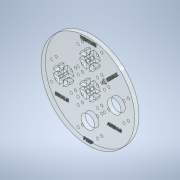
# Autodesk Inventor part: Top_Plate_For_Valve
Saved by Autodesk Inventor 2020 (Build 240168000, 168)
## iProperties
Created: 2021-06-26
Part Number: Top_Plate_For_Valve
Material: Glass
Document SubType Name: Modeling
Designer: Workshop
Density: 2.18 g/cm^3
Appearance: Clear
Author: Workshop
Autodesk Inventor part; units mm, degrees
ref_plane "YZ Plane" through (0, 0, 0) normal (1, 0, 0) x (0, 1, 0)
ref_plane "XZ Plane" through (0, 0, 0) normal (0, 1, 0) x (-1, 0, 0)
ref_plane "XY Plane" through (0, 0, 0) normal (0, 0, 1) x (1, 0, 0)
sketch "Sketch1" plane through (0, 0, 0) normal (0, 0, 1) x (1, 0, 0)
  circle A0 centre (0, -30.9758) radius 8 projected
  circle A1 centre (42.3779, -11.4021) radius 1.5 projected
  circle A2 centre (11.4021, -19.5736) radius 1.5 projected
  circle A3 centre (-11.4021, -19.5737) radius 1.5 projected
  circle A4 centre (-11.4021, -42.3779) radius 1.5 projected
  circle A5 centre (11.4021, -42.3778) radius 1.5 projected
  circle A6 centre (19.5737, -11.4021) radius 1.5 projected
  circle A7 centre (42.3778, 11.4021) radius 1.5 projected
  circle A8 centre (19.5736, 11.4021) radius 1.5 projected
  circle A9 centre (-19.5736, -11.4021) radius 1.5 projected
  circle A10 centre (-11.4021, 11.4021) radius 1.5 projected
  circle A11 centre (0, 0) radius 55 projected
  circle A12 centre (-42.3778, -11.4021) radius 1.5 projected
  circle A13 centre (-11.4021, 19.5736) radius 1.5 projected
  circle A14 centre (11.4021, 19.5737) radius 1.5 projected
  circle A15 centre (-19.5737, 11.4021) radius 1.5 projected
  circle A16 centre (-42.3779, 11.4021) radius 1.5 projected
  line L0 (-3.5186, 28.9238) -> (-9.6538, 28.9238) projected
  arc A17 (-9.6538, 28.9238) -> (-2.019, 21.3151) centre (0, 30.9758) ccw projected
  line L1 (-2.019, 21.3151) -> (-2.0129, 27.4347) projected
  arc A18 (-3.5186, 28.9238) -> (-2.0129, 27.4347) centre (0, 30.9758) ccw projected
  line L2 (3.5186, 28.9238) -> (9.6538, 28.9238) projected
  arc A19 (2.019, 21.3151) -> (9.6538, 28.9238) centre (0, 30.9758) ccw projected
  line L3 (2.019, 21.3151) -> (2.0129, 27.4347) projected
  arc A20 (2.0129, 27.4347) -> (3.5186, 28.9238) centre (0, 30.9758) ccw projected
  line L4 (-3.5186, 33.0277) -> (-9.6538, 33.0277) projected
  arc A21 (-2.019, 40.6365) -> (-9.6538, 33.0277) centre (0, 30.9758) ccw projected
  line L5 (-2.019, 40.6365) -> (-2.0129, 34.5169) projected
  arc A22 (-2.0129, 34.5169) -> (-3.5186, 33.0277) centre (0, 30.9758) ccw projected
  line L6 (3.5186, 33.0277) -> (9.6538, 33.0277) projected
  arc A23 (9.6538, 33.0277) -> (2.019, 40.6365) centre (0, 30.9758) ccw projected
  line L7 (2.019, 40.6365) -> (2.0129, 34.5169) projected
  arc A24 (3.5186, 33.0277) -> (2.0129, 34.5169) centre (0, 30.9758) ccw projected
  circle A25 centre (0, 30.9758) radius 2.25 projected
  circle A26 centre (11.4021, 42.3779) radius 1.5 projected
  circle A27 centre (-11.4021, 42.3778) radius 1.5 projected
  line L8 (-2.052, 3.5186) -> (-2.052, 9.6538) projected
  arc A28 (-2.052, 9.6538) -> (-9.6607, 2.019) centre (0, 0) ccw projected
  line L9 (-9.6607, 2.019) -> (-3.5411, 2.0129) projected
  arc A29 (-2.052, 3.5186) -> (-3.5411, 2.0129) centre (0, 0) ccw projected
  circle A30 centre (0, 0) radius 2.25 projected
  line L10 (-2.052, -3.5186) -> (-2.052, -9.6538) projected
  arc A31 (-9.6607, -2.019) -> (-2.052, -9.6538) centre (0, 0) ccw projected
  line L11 (-9.6607, -2.019) -> (-3.5411, -2.0129) projected
  arc A32 (-3.5411, -2.0129) -> (-2.052, -3.5186) centre (0, 0) ccw projected
  circle A33 centre (-11.4021, -11.4021) radius 1.5 projected
  line L12 (-33.0277, -3.5186) -> (-33.0277, -9.6538) projected
  arc A34 (-40.6365, -2.019) -> (-33.0277, -9.6538) centre (-30.9758, 0) ccw projected
  line L13 (-40.6365, -2.019) -> (-34.5169, -2.0129) projected
  arc A35 (-34.5169, -2.0129) -> (-33.0277, -3.5186) centre (-30.9758, 0) ccw projected
  line L14 (-33.0277, 3.5186) -> (-33.0277, 9.6538) projected
  arc A36 (-33.0277, 9.6538) -> (-40.6365, 2.019) centre (-30.9758, 0) ccw projected
  line L15 (-40.6365, 2.019) -> (-34.5169, 2.0129) projected
  arc A37 (-33.0277, 3.5186) -> (-34.5169, 2.0129) centre (-30.9758, 0) ccw projected
  line L16 (2.052, 3.5186) -> (2.052, 9.6538) projected
  arc A38 (9.6607, 2.019) -> (2.052, 9.6538) centre (0, 0) ccw projected
  line L17 (9.6607, 2.019) -> (3.5411, 2.0129) projected
  arc A39 (3.5411, 2.0129) -> (2.052, 3.5186) centre (0, 0) ccw projected
  line L18 (2.052, -3.5186) -> (2.052, -9.6538) projected
  arc A40 (2.052, -9.6538) -> (9.6607, -2.019) centre (0, 0) ccw projected
  line L19 (9.6607, -2.019) -> (3.5411, -2.0129) projected
  arc A41 (2.052, -3.5186) -> (3.5411, -2.0129) centre (0, 0) ccw projected
  line L20 (-28.9238, 3.5186) -> (-28.9238, 9.6538) projected
  arc A42 (-21.3151, 2.019) -> (-28.9238, 9.6538) centre (-30.9758, 0) ccw projected
  line L21 (-21.3151, 2.019) -> (-27.4347, 2.0129) projected
  arc A43 (-27.4347, 2.0129) -> (-28.9238, 3.5186) centre (-30.9758, 0) ccw projected
  line L22 (-28.9238, -3.5186) -> (-28.9238, -9.6538) projected
  arc A44 (-28.9238, -9.6538) -> (-21.3151, -2.019) centre (-30.9758, 0) ccw projected
  line L23 (-21.3151, -2.019) -> (-27.4347, -2.0129) projected
  arc A45 (-28.9238, -3.5186) -> (-27.4347, -2.0129) centre (-30.9758, 0) ccw projected
  circle A46 centre (-30.9758, 0) radius 1.5 projected
  circle A47 centre (11.4021, 11.4021) radius 1.5 projected
  circle A48 centre (30.9758, 0) radius 8 projected
  circle A49 centre (11.4021, -11.4021) radius 1.5 projected
  point P0 (0, 0)
extrude "Extrusion1" add sketch "Sketch1" along normal mid plane 5
sketch "Sketch2" plane through (0, 0, 2.5) normal (0, 0, 1) x (1, 0, 0)
  line L0 (-9.3534, 52.1011) -> (9.3534, 52.1011) construction
  line L1 (9.3534, 52.1011) -> (9.3534, 49) construction
  line L2 (9.3534, 49) -> (-9.3534, 49) construction
  line L3 (-9.3534, 49) -> (-9.3534, 52.1011) construction
  line L4 (-38.9076, -20) -> (-23.0439, -20) construction
  line L5 (-23.0439, -20) -> (-23.0439, -23.05) construction
  line L6 (-23.0439, -23.05) -> (-38.9076, -23.05) construction
  line L7 (-38.9076, -23.05) -> (-38.9076, -20) construction
  line L8 (22.3314, -20) -> (39.6201, -20) construction
  line L9 (39.6201, -20) -> (39.6201, -23.05) construction
  line L10 (39.6201, -23.05) -> (22.3314, -23.05) construction
  line L11 (22.3314, -23.05) -> (22.3314, -20) construction
  line L12 (-5.6862, -49) -> (5.6862, -49) construction
  line L13 (5.6862, -49) -> (5.6862, -52.05) construction
  line L14 (5.6862, -52.05) -> (-5.6862, -52.05) construction
  line L15 (-5.6862, -52.05) -> (-5.6862, -49) construction
  line L16 (20.842, 22.9986) -> (33.067, 35.2236) construction
  line L17 (33.067, 35.2236) -> (35.2236, 33.067) construction
  line L18 (35.2236, 33.067) -> (22.9986, 20.842) construction
  line L19 (22.9986, 20.842) -> (20.842, 22.9986) construction
  circle A0 centre (-30.9758, 0) radius 1.5 projected
  circle A1 centre (30.9758, 0) radius 8 projected
  circle A2 centre (0, 0) radius 2.25 projected
  line L20 (0, 0) -> (21.9203, 21.9203) construction
  line L21 (0, 0) -> (31, 0) construction
  line L22 (-8.2631, 49.0511) -> (-9.3534, 52.1011)
  line L23 (-9.3534, 52.1011) -> (-8.6862, 52.1011)
  line L24 (-8.6862, 52.1011) -> (-7.9121, 49.8439)
  line L25 (-7.9121, 49.8439) -> (-7.1659, 52.1011)
  line L26 (-7.1659, 52.1011) -> (-6.5126, 52.1011)
  line L27 (-6.5126, 52.1011) -> (-7.6029, 49.0511)
  line L28 (-7.6029, 49.0511) -> (-8.2631, 49.0511)
  line L29 (-6.1988, 49.0511) -> (-6.1988, 52.1011)
  line L30 (-6.1988, 52.1011) -> (-3.9369, 52.1011)
  line L31 (-3.9369, 52.1011) -> (-3.9369, 51.5851)
  line L32 (-3.9369, 51.5851) -> (-5.5828, 51.5851)
  line L33 (-5.5828, 51.5851) -> (-5.5828, 50.9086)
  line L34 (-5.5828, 50.9086) -> (-4.0508, 50.9086)
  line L35 (-4.0508, 50.9086) -> (-4.0508, 50.3925)
  line L36 (-4.0508, 50.3925) -> (-5.5828, 50.3925)
  line L37 (-5.5828, 50.3925) -> (-5.5828, 49.5672)
  line L38 (-5.5828, 49.5672) -> (-3.8788, 49.5672)
  line L39 (-3.8788, 49.5672) -> (-3.8788, 49.0511)
  line L40 (-3.8788, 49.0511) -> (-6.1988, 49.0511)
  line L41 (-3.351, 49.0511) -> (-3.351, 52.1011)
  line L42 (-3.351, 52.1011) -> (-2.7536, 52.1011)
  line L43 (-2.7536, 52.1011) -> (-1.5006, 50.0554)
  line L44 (-1.5006, 50.0554) -> (-1.5006, 52.1011)
  line L45 (-1.5006, 52.1011) -> (-0.931, 52.1011)
  line L46 (-0.931, 52.1011) -> (-0.931, 49.0511)
  line L47 (-0.931, 49.0511) -> (-1.5471, 49.0511)
  line L48 (-1.5471, 49.0511) -> (-2.7815, 51.0527)
  line L49 (-2.7815, 51.0527) -> (-2.7815, 49.0511)
  line L50 (-2.7815, 49.0511) -> (-3.351, 49.0511)
  line L51 (0.408, 49.0511) -> (0.408, 51.5851)
  line L52 (0.408, 51.5851) -> (-0.4963, 51.5851)
  line L53 (-0.4963, 51.5851) -> (-0.4963, 52.1011)
  line L54 (-0.4963, 52.1011) -> (1.926, 52.1011)
  line L55 (1.926, 52.1011) -> (1.926, 51.5851)
  line L56 (1.926, 51.5851) -> (1.024, 51.5851)
  line L57 (1.024, 51.5851) -> (1.024, 49.0511)
  line L58 (1.024, 49.0511) -> (0.408, 49.0511)
  line L59 (2.3212, 52.1011) -> (2.9373, 52.1011)
  line L60 (2.9373, 52.1011) -> (2.9373, 50.4483)
  spline S0 degree 2 poles (2.9373, 50.4483) (2.9373, 50.0554) (2.9605, 49.9392) knots 0 0 0 1 1 1
  spline S1 degree 2 poles (2.9605, 49.9392) (3, 49.7532) (3.2976, 49.5254) (3.5556, 49.5254) knots 0 0 0 1 2 2 2
  spline S2 degree 2 poles (3.5556, 49.5254) (3.816, 49.5254) (4.0833, 49.7393) (4.1368, 50.0508) (4.1368, 50.4134) knots 0 0 0 1 2 3 3 3
  line L61 (4.1368, 50.4134) -> (4.1368, 52.1011)
  line L62 (4.1368, 52.1011) -> (4.7528, 52.1011)
  line L63 (4.7528, 52.1011) -> (4.7528, 50.4994)
  spline S3 degree 2 poles (4.7528, 50.4994) (4.7528, 49.9508) (4.6529, 49.4975) (4.3855, 49.186) (3.9345, 49) (3.5742, 49) knots 0 0 0 1 2 3 4 4 4
  spline S4 degree 2 poles (3.5742, 49) (3.1372, 49) (2.6862, 49.2022) (2.4235, 49.5231) (2.3817, 49.7021) knots 0 0 0 1 2 3 3 3
  spline S5 degree 2 poles (2.3817, 49.7021) (2.3212, 49.9624) (2.3212, 50.4739) knots 0 0 0 1 1 1
  line L64 (2.3212, 50.4739) -> (2.3212, 52.1011)
  line L65 (5.4038, 49.0511) -> (5.4038, 52.1011)
  line L66 (5.4038, 52.1011) -> (6.7009, 52.1011)
  spline S6 degree 2 poles (6.7009, 52.1011) (7.1914, 52.1011) (7.6331, 51.9361) (7.9005, 51.5176) (7.9005, 51.2457) knots 0 0 0 1 2 3 3 3
  spline S7 degree 2 poles (7.9005, 51.2457) (7.9005, 50.9039) (7.4983, 50.4553) (7.0961, 50.3971) knots 0 0 0 1 2 2 2
  spline S8 degree 2 poles (7.0961, 50.3971) (7.2961, 50.2809) (7.5564, 50.0019) (7.7773, 49.6463) knots 0 0 0 1 2 2 2
  line L67 (7.7773, 49.6463) -> (8.1492, 49.0511)
  line L68 (8.1492, 49.0511) -> (7.4123, 49.0511)
  line L69 (7.4123, 49.0511) -> (6.9683, 49.716)
  spline S9 degree 2 poles (6.9683, 49.716) (6.7288, 50.0717) (6.5545, 50.2577) (6.3592, 50.3251) (6.1453, 50.3251) knots 0 0 0 1 2 3 3 3
  line L70 (6.1453, 50.3251) -> (6.0198, 50.3251)
  line L71 (6.0198, 50.3251) -> (6.0198, 49.0511)
  line L72 (6.0198, 49.0511) -> (5.4038, 49.0511)
  line L73 (6.0198, 50.8109) -> (6.4754, 50.8109)
  spline S10 degree 2 poles (6.4754, 50.8109) (6.9195, 50.8109) (7.1403, 50.8853) (7.2658, 51.069) (7.2658, 51.2061) knots 0 0 0 1 2 3 3 3
  spline S11 degree 2 poles (7.2658, 51.2061) (7.2658, 51.3596) (7.1008, 51.5502) (6.952, 51.5758) knots 0 0 0 1 2 2 2
  spline S12 degree 2 poles (6.952, 51.5758) (6.8753, 51.5851) (6.501, 51.5851) knots 0 0 0 1 1 1
  line L74 (6.501, 51.5851) -> (6.0198, 51.5851)
  line L75 (6.0198, 51.5851) -> (6.0198, 50.8109)
  line L76 (8.4607, 49.0511) -> (8.4607, 52.1011)
  line L77 (8.4607, 52.1011) -> (9.0768, 52.1011)
  line L78 (9.0768, 52.1011) -> (9.0768, 49.0511)
  line L79 (9.0768, 49.0511) -> (8.4607, 49.0511)
  line L80 (23.2189, 21.0622) -> (21.0622, 23.2189)
  line L81 (21.0622, 23.2189) -> (22.6617, 24.8183)
  line L82 (22.6617, 24.8183) -> (23.0266, 24.4534)
  line L83 (23.0266, 24.4534) -> (21.8628, 23.2896)
  line L84 (21.8628, 23.2896) -> (22.3411, 22.8113)
  line L85 (22.3411, 22.8113) -> (23.4244, 23.8945)
  line L86 (23.4244, 23.8945) -> (23.7893, 23.5296)
  line L87 (23.7893, 23.5296) -> (22.7061, 22.4463)
  line L88 (22.7061, 22.4463) -> (23.2896, 21.8628)
  line L89 (23.2896, 21.8628) -> (24.4945, 23.0677)
  line L90 (24.4945, 23.0677) -> (24.8594, 22.7028)
  line L91 (24.8594, 22.7028) -> (23.2189, 21.0622)
  line L92 (25.0107, 22.854) -> (24.6326, 24.7214)
  line L93 (24.6326, 24.7214) -> (22.923, 25.0797)
  line L94 (22.923, 25.0797) -> (23.431, 25.5876)
  line L95 (23.431, 25.5876) -> (24.5027, 25.3707)
  line L96 (24.5027, 25.3707) -> (24.2857, 26.4424)
  line L97 (24.2857, 26.4424) -> (24.7937, 26.9504)
  line L98 (24.7937, 26.9504) -> (25.1471, 25.2392)
  line L99 (25.1471, 25.2392) -> (27.0161, 24.8594)
  line L100 (27.0161, 24.8594) -> (26.4901, 24.3334)
  line L101 (26.4901, 24.3334) -> (25.2819, 24.5849)
  line L102 (25.2819, 24.5849) -> (25.5334, 23.3767)
  line L103 (25.5334, 23.3767) -> (25.0107, 22.854)
  line L104 (27.2397, 25.083) -> (25.083, 27.2397)
  line L105 (25.083, 27.2397) -> (25.5186, 27.6753)
  line L106 (25.5186, 27.6753) -> (26.3668, 26.8271)
  line L107 (26.3668, 26.8271) -> (27.2199, 27.6802)
  line L108 (27.2199, 27.6802) -> (26.3717, 28.5284)
  line L109 (26.3717, 28.5284) -> (26.8074, 28.964)
  line L110 (26.8074, 28.964) -> (28.964, 26.8074)
  line L111 (28.964, 26.8074) -> (28.5284, 26.3717)
  line L112 (28.5284, 26.3717) -> (27.5849, 27.3153)
  line L113 (27.5849, 27.3153) -> (26.7317, 26.4622)
  line L114 (26.7317, 26.4622) -> (27.6753, 25.5186)
  line L115 (27.6753, 25.5186) -> (27.2397, 25.083)
  line L116 (31.3591, 29.2024) -> (30.8856, 28.729)
  line L117 (30.8856, 28.729) -> (30.2084, 29.0314)
  line L118 (30.2084, 29.0314) -> (29.347, 28.1701)
  line L119 (29.347, 28.1701) -> (29.6577, 27.501)
  line L120 (29.6577, 27.501) -> (29.1958, 27.0391)
  line L121 (29.1958, 27.0391) -> (27.8775, 30.0341)
  line L122 (27.8775, 30.0341) -> (28.341, 30.4977)
  line L123 (28.341, 30.4977) -> (31.3591, 29.2024)
  line L124 (29.7037, 29.2566) -> (28.6073, 29.758)
  line L125 (28.6073, 29.758) -> (29.1136, 28.6665)
  line L126 (29.1136, 28.6665) -> (29.7037, 29.2566)
  line L127 (31.604, 29.4473) -> (29.4654, 31.5859)
  line L128 (29.4654, 31.5859) -> (29.901, 32.0215)
  line L129 (29.901, 32.0215) -> (31.6747, 30.2478)
  line L130 (31.6747, 30.2478) -> (32.7579, 31.3311)
  line L131 (32.7579, 31.3311) -> (33.1229, 30.9662)
  line L132 (33.1229, 30.9662) -> (31.604, 29.4473)
  line L133 (33.4335, 31.2769) -> (31.2769, 33.4335)
  line L134 (31.2769, 33.4335) -> (32.8763, 35.033)
  line L135 (32.8763, 35.033) -> (33.2412, 34.668)
  line L136 (33.2412, 34.668) -> (32.0774, 33.5042)
  line L137 (32.0774, 33.5042) -> (32.5557, 33.0259)
  line L138 (32.5557, 33.0259) -> (33.639, 34.1091)
  line L139 (33.639, 34.1091) -> (34.0039, 33.7442)
  line L140 (34.0039, 33.7442) -> (32.9207, 32.6609)
  line L141 (32.9207, 32.6609) -> (33.5042, 32.0774)
  line L142 (33.5042, 32.0774) -> (34.7091, 33.2823)
  line L143 (34.7091, 33.2823) -> (35.0741, 32.9174)
  line L144 (35.0741, 32.9174) -> (33.4335, 31.2769)
  line L145 (25.3907, -23.1011) -> (24.7212, -23.1011)
  line L146 (24.7212, -23.1011) -> (24.4562, -22.4084)
  line L147 (24.4562, -22.4084) -> (23.238, -22.4084)
  line L148 (23.238, -22.4084) -> (22.9846, -23.1011)
  line L149 (22.9846, -23.1011) -> (22.3314, -23.1011)
  line L150 (22.3314, -23.1011) -> (23.517, -20.0511)
  line L151 (23.517, -20.0511) -> (24.1725, -20.0511)
  line L152 (24.1725, -20.0511) -> (25.3907, -23.1011)
  line L153 (24.2586, -21.8923) -> (23.8378, -20.7625)
  line L154 (23.8378, -20.7625) -> (23.424, -21.8923)
  line L155 (23.424, -21.8923) -> (24.2586, -21.8923)
  line L156 (25.6999, -23.1011) -> (25.6999, -20.0511)
  line L157 (25.6999, -20.0511) -> (26.3159, -20.0511)
  line L158 (26.3159, -20.0511) -> (26.3159, -23.1011)
  line L159 (26.3159, -23.1011) -> (25.6999, -23.1011)
  line L160 (26.9041, -23.1011) -> (26.9041, -20.0511)
  line L161 (26.9041, -20.0511) -> (28.2012, -20.0511)
  spline S13 degree 2 poles (28.2012, -20.0511) (28.6918, -20.0511) (29.1334, -20.2162) (29.4008, -20.6346) (29.4008, -20.9066) knots 0 0 0 1 2 3 3 3
  spline S14 degree 2 poles (29.4008, -20.9066) (29.4008, -21.2484) (28.9986, -21.697) (28.5964, -21.7551) knots 0 0 0 1 2 2 2
  spline S15 degree 2 poles (28.5964, -21.7551) (28.7964, -21.8714) (29.0567, -22.1503) (29.2776, -22.506) knots 0 0 0 1 2 2 2
  line L162 (29.2776, -22.506) -> (29.6495, -23.1011)
  line L163 (29.6495, -23.1011) -> (28.9126, -23.1011)
  line L164 (28.9126, -23.1011) -> (28.4686, -22.4363)
  spline S16 degree 2 poles (28.4686, -22.4363) (28.2291, -22.0806) (28.0548, -21.8946) (27.8595, -21.8272) (27.6456, -21.8272) knots 0 0 0 1 2 3 3 3
  line L165 (27.6456, -21.8272) -> (27.5201, -21.8272)
  line L166 (27.5201, -21.8272) -> (27.5201, -23.1011)
  line L167 (27.5201, -23.1011) -> (26.9041, -23.1011)
  line L168 (27.5201, -21.3413) -> (27.9757, -21.3413)
  spline S17 degree 2 poles (27.9757, -21.3413) (28.4198, -21.3413) (28.6406, -21.267) (28.7661, -21.0833) (28.7661, -20.9462) knots 0 0 0 1 2 3 3 3
  spline S18 degree 2 poles (28.7661, -20.9462) (28.7661, -20.7927) (28.6011, -20.6021) (28.4523, -20.5765) knots 0 0 0 1 2 2 2
  spline S19 degree 2 poles (28.4523, -20.5765) (28.3756, -20.5672) (28.0013, -20.5672) knots 0 0 0 1 1 1
  line L169 (28.0013, -20.5672) -> (27.5201, -20.5672)
  line L170 (27.5201, -20.5672) -> (27.5201, -21.3413)
  line L171 (29.982, -20.0511) -> (31.2024, -20.0511)
  spline S20 degree 2 poles (31.2024, -20.0511) (31.5651, -20.0511) (31.9208, -20.1116) (32.202, -20.3022) (32.3903, -20.6207) (32.3903, -20.8183) knots 0 0 0 1 2 3 4 4 4
  spline S21 degree 2 poles (32.3903, -20.8183) (32.3903, -21.0322) (32.1602, -21.3878) (31.9626, -21.4785) knots 0 0 0 1 2 2 2
  spline S22 degree 2 poles (31.9626, -21.4785) (32.2416, -21.5599) (32.5391, -21.9504) (32.5391, -22.2154) knots 0 0 0 1 2 2 2
  spline S23 degree 2 poles (32.5391, -22.2154) (32.5391, -22.4247) (32.3462, -22.8175) (32.0091, -23.0523) (31.765, -23.0802) knots 0 0 0 1 2 3 3 3
  spline S24 degree 2 poles (31.765, -23.0802) (31.6092, -23.0965) (31.0211, -23.1011) knots 0 0 0 1 1 1
  line L172 (31.0211, -23.1011) -> (29.982, -23.1011)
  line L173 (29.982, -23.1011) -> (29.982, -20.0511)
  line L174 (30.598, -21.7691) -> (30.598, -22.5851)
  line L175 (30.598, -22.5851) -> (31.1699, -22.5851)
  spline S25 degree 2 poles (31.1699, -22.5851) (31.5046, -22.5851) (31.593, -22.5665) knots 0 0 0 1 1 1
  spline S26 degree 2 poles (31.593, -22.5665) (31.7301, -22.5409) (31.9045, -22.3479) (31.9045, -22.1852) knots 0 0 0 1 2 2 2
  spline S27 degree 2 poles (31.9045, -22.1852) (31.9045, -22.0481) (31.772, -21.8574) (31.5186, -21.7691) (31.0978, -21.7691) knots 0 0 0 1 2 3 3 3
  line L176 (31.0978, -21.7691) -> (30.598, -21.7691)
  line L177 (30.598, -20.5579) -> (30.598, -21.2623)
  line L178 (30.598, -21.2623) -> (31.0025, -21.2623)
  spline S28 degree 2 poles (31.0025, -21.2623) (31.3628, -21.2623) (31.4512, -21.253) knots 0 0 0 1 1 1
  spline S29 degree 2 poles (31.4512, -21.253) (31.6092, -21.2321) (31.7906, -21.0531) (31.7906, -20.9043) knots 0 0 0 1 2 2 2
  spline S30 degree 2 poles (31.7906, -20.9043) (31.7906, -20.7625) (31.6348, -20.5881) (31.4791, -20.5672) knots 0 0 0 1 2 2 2
  spline S31 degree 2 poles (31.4791, -20.5672) (31.3884, -20.5579) (30.9514, -20.5579) knots 0 0 0 1 1 1
  line L179 (30.9514, -20.5579) -> (30.598, -20.5579)
  line L180 (35.8076, -23.1011) -> (35.1381, -23.1011)
  line L181 (35.1381, -23.1011) -> (34.8731, -22.4084)
  line L182 (34.8731, -22.4084) -> (33.655, -22.4084)
  line L183 (33.655, -22.4084) -> (33.4016, -23.1011)
  line L184 (33.4016, -23.1011) -> (32.7483, -23.1011)
  line L185 (32.7483, -23.1011) -> (33.9339, -20.0511)
  line L186 (33.9339, -20.0511) -> (34.5895, -20.0511)
  line L187 (34.5895, -20.0511) -> (35.8076, -23.1011)
  line L188 (34.6755, -21.8923) -> (34.2547, -20.7625)
  line L189 (34.2547, -20.7625) -> (33.841, -21.8923)
  line L190 (33.841, -21.8923) -> (34.6755, -21.8923)
  line L191 (37.5558, -21.983) -> (37.5558, -21.4669)
  line L192 (37.5558, -21.4669) -> (38.8832, -21.4669)
  line L193 (38.8832, -21.4669) -> (38.8832, -22.6804)
  spline S32 degree 2 poles (38.8832, -22.6804) (38.6903, -22.8687) (37.9557, -23.1523) (37.5791, -23.1523) knots 0 0 0 1 2 2 2
  spline S33 degree 2 poles (37.5791, -23.1523) (37.1002, -23.1523) (36.3888, -22.7501) (36.0308, -22.0039) (36.0308, -21.5668) knots 0 0 0 1 2 3 3 3
  spline S34 degree 2 poles (36.0308, -21.5668) (36.0308, -21.0903) (36.4307, -20.3487) (36.8142, -20.1511) knots 0 0 0 1 2 2 2
  spline S35 degree 2 poles (36.8142, -20.1511) (37.1095, -20) (37.5465, -20) knots 0 0 0 1 1 1
  spline S36 degree 2 poles (37.5465, -20) (38.1137, -20) (38.753, -20.4766) (38.8437, -20.8973) knots 0 0 0 1 2 2 2
  line L194 (38.8437, -20.8973) -> (38.2323, -21.0112)
  spline S37 degree 2 poles (38.2323, -21.0112) (38.1672, -20.7857) (37.8115, -20.5254) (37.5465, -20.5254) knots 0 0 0 1 2 2 2
  spline S38 degree 2 poles (37.5465, -20.5254) (37.142, -20.5254) (36.6655, -21.0368) (36.6655, -21.5413) knots 0 0 0 1 2 2 2
  spline S39 degree 2 poles (36.6655, -21.5413) (36.6655, -22.0829) (37.149, -22.6269) (37.5395, -22.6269) knots 0 0 0 1 2 2 2
  spline S40 degree 2 poles (37.5395, -22.6269) (37.7325, -22.6269) (38.1207, -22.4758) (38.2602, -22.3689) knots 0 0 0 1 2 2 2
  line L195 (38.2602, -22.3689) -> (38.2602, -21.983)
  line L196 (38.2602, -21.983) -> (37.5558, -21.983)
  line L197 (-5.3747, -52.05) -> (-5.3747, -49)
  line L198 (-5.3747, -49) -> (-4.3867, -49)
  spline S41 degree 2 poles (-4.3867, -49) (-3.8241, -49) (-3.6544, -49.0465) knots 0 0 0 1 1 1
  spline S42 degree 2 poles (-3.6544, -49.0465) (-3.3917, -49.1139) (-3.0384, -49.5742) (-3.0384, -49.9392) knots 0 0 0 1 2 2 2
  spline S43 degree 2 poles (-3.0384, -49.9392) (-3.0384, -50.2181) (-3.2429, -50.6017) (-3.5568, -50.8202) (-3.7195, -50.8551) knots 0 0 0 1 2 3 3 3
  spline S44 degree 2 poles (-3.7195, -50.8551) (-3.938, -50.8993) (-4.3565, -50.8993) knots 0 0 0 1 1 1
  line L199 (-4.3565, -50.8993) -> (-4.7587, -50.8993)
  line L200 (-4.7587, -50.8993) -> (-4.7587, -52.05)
  line L201 (-4.7587, -52.05) -> (-5.3747, -52.05)
  line L202 (-4.7587, -49.5161) -> (-4.7587, -50.3832)
  line L203 (-4.7587, -50.3832) -> (-4.4216, -50.3832)
  spline S45 degree 2 poles (-4.4216, -50.3832) (-4.0566, -50.3832) (-3.8125, -50.2879) (-3.673, -50.0833) (-3.673, -49.9485) knots 0 0 0 1 2 3 3 3
  spline S46 degree 2 poles (-3.673, -49.9485) (-3.673, -49.7811) (-3.8683, -49.5649) (-4.0194, -49.537) knots 0 0 0 1 2 2 2
  spline S47 degree 2 poles (-4.0194, -49.537) (-4.1287, -49.5161) (-4.4611, -49.5161) knots 0 0 0 1 1 1
  line L204 (-4.4611, -49.5161) -> (-4.7587, -49.5161)
  line L205 (-2.5316, -52.05) -> (-2.5316, -49)
  line L206 (-2.5316, -49) -> (-0.2697, -49)
  line L207 (-0.2697, -49) -> (-0.2697, -49.5161)
  line L208 (-0.2697, -49.5161) -> (-1.9155, -49.5161)
  line L209 (-1.9155, -49.5161) -> (-1.9155, -50.1926)
  line L210 (-1.9155, -50.1926) -> (-0.3836, -50.1926)
  line L211 (-0.3836, -50.1926) -> (-0.3836, -50.7087)
  line L212 (-0.3836, -50.7087) -> (-1.9155, -50.7087)
  line L213 (-1.9155, -50.7087) -> (-1.9155, -51.5339)
  line L214 (-1.9155, -51.5339) -> (-0.2115, -51.5339)
  line L215 (-0.2115, -51.5339) -> (-0.2115, -52.05)
  line L216 (-0.2115, -52.05) -> (-2.5316, -52.05)
  line L217 (0.3115, -52.05) -> (0.3115, -49)
  line L218 (0.3115, -49) -> (2.5734, -49)
  line L219 (2.5734, -49) -> (2.5734, -49.5161)
  line L220 (2.5734, -49.5161) -> (0.9276, -49.5161)
  line L221 (0.9276, -49.5161) -> (0.9276, -50.1926)
  line L222 (0.9276, -50.1926) -> (2.4595, -50.1926)
  line L223 (2.4595, -50.1926) -> (2.4595, -50.7087)
  line L224 (2.4595, -50.7087) -> (0.9276, -50.7087)
  line L225 (0.9276, -50.7087) -> (0.9276, -51.5339)
  line L226 (0.9276, -51.5339) -> (2.6316, -51.5339)
  line L227 (2.6316, -51.5339) -> (2.6316, -52.05)
  line L228 (2.6316, -52.05) -> (0.3115, -52.05)
  line L229 (3.1546, -52.05) -> (3.1546, -49)
  line L230 (3.1546, -49) -> (4.1426, -49)
  spline S48 degree 2 poles (4.1426, -49) (4.7052, -49) (4.8749, -49.0465) knots 0 0 0 1 1 1
  spline S49 degree 2 poles (4.8749, -49.0465) (5.1376, -49.1139) (5.4909, -49.5742) (5.4909, -49.9392) knots 0 0 0 1 2 2 2
  spline S50 degree 2 poles (5.4909, -49.9392) (5.4909, -50.2181) (5.2864, -50.6017) (4.9725, -50.8202) (4.8098, -50.8551) knots 0 0 0 1 2 3 3 3
  spline S51 degree 2 poles (4.8098, -50.8551) (4.5913, -50.8993) (4.1728, -50.8993) knots 0 0 0 1 1 1
  line L231 (4.1728, -50.8993) -> (3.7707, -50.8993)
  line L232 (3.7707, -50.8993) -> (3.7707, -52.05)
  line L233 (3.7707, -52.05) -> (3.1546, -52.05)
  line L234 (3.7707, -49.5161) -> (3.7707, -50.3832)
  line L235 (3.7707, -50.3832) -> (4.1077, -50.3832)
  spline S52 degree 2 poles (4.1077, -50.3832) (4.4727, -50.3832) (4.7168, -50.2879) (4.8563, -50.0833) (4.8563, -49.9485) knots 0 0 0 1 2 3 3 3
  spline S53 degree 2 poles (4.8563, -49.9485) (4.8563, -49.7811) (4.661, -49.5649) (4.5099, -49.537) knots 0 0 0 1 2 2 2
  spline S54 degree 2 poles (4.5099, -49.537) (4.4006, -49.5161) (4.0682, -49.5161) knots 0 0 0 1 1 1
  line L236 (4.0682, -49.5161) -> (3.7707, -49.5161)
  line L237 (-38.617, -23.05) -> (-38.617, -20)
  line L238 (-38.617, -20) -> (-38.001, -20)
  line L239 (-38.001, -20) -> (-38.001, -23.05)
  line L240 (-38.001, -23.05) -> (-38.617, -23.05)
  line L241 (-37.4082, -23.05) -> (-37.4082, -20)
  line L242 (-37.4082, -20) -> (-36.8108, -20)
  line L243 (-36.8108, -20) -> (-35.5577, -22.0457)
  line L244 (-35.5577, -22.0457) -> (-35.5577, -20)
  line L245 (-35.5577, -20) -> (-34.9882, -20)
  line L246 (-34.9882, -20) -> (-34.9882, -23.05)
  line L247 (-34.9882, -23.05) -> (-35.6042, -23.05)
  line L248 (-35.6042, -23.05) -> (-36.8386, -21.0484)
  line L249 (-36.8386, -21.0484) -> (-36.8386, -23.05)
  line L250 (-36.8386, -23.05) -> (-37.4082, -23.05)
  line L251 (-34.335, -23.05) -> (-34.335, -20)
  line L252 (-34.335, -20) -> (-33.7189, -20)
  line L253 (-33.7189, -20) -> (-33.7189, -21.1995)
  line L254 (-33.7189, -21.1995) -> (-32.5124, -21.1995)
  line L255 (-32.5124, -21.1995) -> (-32.5124, -20)
  line L256 (-32.5124, -20) -> (-31.8963, -20)
  line L257 (-31.8963, -20) -> (-31.8963, -23.05)
  line L258 (-31.8963, -23.05) -> (-32.5124, -23.05)
  line L259 (-32.5124, -23.05) -> (-32.5124, -21.7156)
  line L260 (-32.5124, -21.7156) -> (-33.7189, -21.7156)
  line L261 (-33.7189, -21.7156) -> (-33.7189, -23.05)
  line L262 (-33.7189, -23.05) -> (-34.335, -23.05)
  line L263 (-28.5093, -23.05) -> (-29.1788, -23.05)
  line L264 (-29.1788, -23.05) -> (-29.4438, -22.3572)
  line L265 (-29.4438, -22.3572) -> (-30.6619, -22.3572)
  line L266 (-30.6619, -22.3572) -> (-30.9153, -23.05)
  line L267 (-30.9153, -23.05) -> (-31.5686, -23.05)
  line L268 (-31.5686, -23.05) -> (-30.383, -20)
  line L269 (-30.383, -20) -> (-29.7274, -20)
  line L270 (-29.7274, -20) -> (-28.5093, -23.05)
  line L271 (-29.6414, -21.8412) -> (-30.0622, -20.7114)
  line L272 (-30.0622, -20.7114) -> (-30.476, -21.8412)
  line L273 (-30.476, -21.8412) -> (-29.6414, -21.8412)
  line L274 (-28.1629, -23.05) -> (-28.1629, -20.0256)
  line L275 (-28.1629, -20.0256) -> (-27.5468, -20.0256)
  line L276 (-27.5468, -20.0256) -> (-27.5468, -22.5339)
  line L277 (-27.5468, -22.5339) -> (-26.0149, -22.5339)
  line L278 (-26.0149, -22.5339) -> (-26.0149, -23.05)
  line L279 (-26.0149, -23.05) -> (-28.1629, -23.05)
  line L280 (-25.5755, -23.05) -> (-25.5755, -20)
  line L281 (-25.5755, -20) -> (-23.3136, -20)
  line L282 (-23.3136, -20) -> (-23.3136, -20.5161)
  line L283 (-23.3136, -20.5161) -> (-24.9595, -20.5161)
  line L284 (-24.9595, -20.5161) -> (-24.9595, -21.1926)
  line L285 (-24.9595, -21.1926) -> (-23.4275, -21.1926)
  line L286 (-23.4275, -21.1926) -> (-23.4275, -21.7087)
  line L287 (-23.4275, -21.7087) -> (-24.9595, -21.7087)
  line L288 (-24.9595, -21.7087) -> (-24.9595, -22.5339)
  line L289 (-24.9595, -22.5339) -> (-23.2555, -22.5339)
  line L290 (-23.2555, -22.5339) -> (-23.2555, -23.05)
  line L291 (-23.2555, -23.05) -> (-25.5755, -23.05)
  point P0 (0, 0)
  point P1 (0, 49)
  point P2 (-30.9758, -20)
  point P3 (30.9758, -20)
  point P4 (0, -49)
  dimension "d10" = 30
  dimension "d11" = 45
  dimension "d12" = 5.25
  dimension "d13" = 5
  dimension "d14" = 23
  dimension "d2" = 49
  dimension "d3" = 49
  dimension "d4" = 20
  dimension "d5" = 20
  dimension "d6" = 31
  dimension "d7" = 45
  constraints: 5 midpoint, 4 end point, 4 vertical alignment, 1 equal length, 1 horizontal, 10 other
  measures "d2" distance of point (0, 49) point (0, 0)
  measures "d3" distance of point (0, 0) point (0, -49)
  measures "d4" distance of A0.centre point (-30.976, -20)
  measures "d5" distance of A1.centre point (30.976, -20)
  measures "d6" distance of L20.end L20.start
  measures "d7" angle of L21 L20
emboss "Emboss1" sketch "Sketch2" operation cut depth 1 direction (0, 0, -1) contours L22 L23 L24 L25 L26 L27 L28 | L29 L30 L31 L32 L33 L34 L35 L36 L37 L38 L39 L40 | L41 L42 L43 L44 L45 L46 L47 L48 L49 L50 | L51 L52 L53 L54 L55 L56 L57 L58 | L59 L60 S0 S1 S2 L61 L62 L63 S3 S4 S5 L64 | L65 L66 S6 S7 S8 L67 L68 L69 S9 L70 L71 L72 | L76 L77 L78 L79 | L80 L81 L82 L83 L84 L85 L86 L87 L88 L89 L90 L91 | L92 L93 L94 L95 L96 L97 L98 L99 L100 L101 L102 L103 | L104 L105 L106 L107 L108 L109 L110 L111 L112 L113 L114 L115 | L116 L117 L118 L119 L120 L121 L122 L123 | L127 L128 L129 L130 L131 L132 | L133 L134 L135 L136 L137 L138 L139 L140 L141 L142 L143 L144 | L145 L146 L147 L148 L149 L150 L151 L152 | L156 L157 L158 L159 | L160 L161 S13 S14 S15 L162 L163 L164 S16 L165 L166 L167 | L171 S20 S21 S22 S23 S24 L172 L173 | L180 L181 L182 L183 L184 L185 L186 L187 | L191 L192 L193 S32 S33 S34 S35 S36 L194 S37 S38 S39 S40 L195 L196 | L197 L198 S41 S42 S43 S44 L199 L200 L201 | L205 L206 L207 L208 L209 L210 L211 L212 L213 L214 L215 L216 | L217 L218 L219 L220 L221 L222 L223 L224 L225 L226 L227 L228 | L229 L230 S48 S49 S50 S51 L231 L232 L233 | L237 L238 L239 L240 | L241 L242 L243 L244 L245 L246 L247 L248 L249 L250 | L251 L252 L253 L254 L255 L256 L257 L258 L259 L260 L261 L262 | L263 L264 L265 L266 L267 L268 L269 L270 | L274 L275 L276 L277 L278 L279 | L280 L281 L282 L283 L284 L285 L286 L287 L288 L289 L290 L291
sketch "Sketch3" plane through (0, 0, 2.5) normal (0, 0, 1) x (1, 0, 0)
  circle A0 centre (0, 0) radius 2.25 projected
  line L0 (0, 0) -> (21.2132, 21.2132) construction
  line L1 (0, 0) -> (30, 0) construction
  line L2 (16.2635, 16.2635) -> (17.7601, 21.2956)
  line L3 (17.7601, 21.2956) -> (21.2956, 17.7601)
  line L4 (21.2956, 17.7601) -> (16.2635, 16.2635)
  point P0 (0, 0)
  point P1 (19.5278, 19.5278)
  dimension "d10" = 30
  dimension "d11" = 45
  dimension "d12" = 5.25
  dimension "d13" = 5
  dimension "d14" = 23
  constraints: 10 end point, 2 equal length, 2 point on line, 1 horizontal, 1 midpoint
  measures "d10" distance of L0.start L0.end
  measures "d11" angle of L1 L0
  measures "d12" distance of L3.end L2.start
  measures "d13" distance of L2.end L3.end
  measures "d14" distance of L0.start L2.start
extrude "Extrusion2" cut sketch "Sketch3" against normal blind 1 contours L2 L3 L4
body "Solid1"
